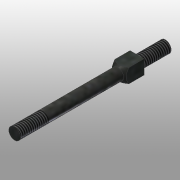
# Autodesk Inventor part: 500-001
Saved by Autodesk Inventor 2016 (Build 200138000, 138)
## iProperties
Created: 2015-04-18
Part Number: 500-001
Material: Steel
Document SubType Name: Modeling
Designer: Station9
Density: 7.85 g/cm^3
Appearance: Plate
Mass: 1.35592 g
Surface Area: 2.8236 cm^2
Volume: 0.172728 cm^3
Author: Station9
Autodesk Inventor part; units mm, degrees
ref_plane "YZ Plane" through (0, 0, 0) normal (1, 0, 0) x (0, 1, 0)
ref_plane "XZ Plane" through (0, 0, 0) normal (0, 1, 0) x (-1, 0, 0)
ref_plane "XY Plane" through (0, 0, 0) normal (0, 0, 1) x (1, 0, 0)
sketch "Sketch1" plane through (0, 0, 0) normal (0, 1, 0) x (-1, 0, 0)
  line L0 (-1.5, 1.5) -> (1.5, 1.5)
  line L1 (1.5, 1.5) -> (1.5, -1.5)
  line L2 (1.5, -1.5) -> (-1.5, -1.5)
  line L3 (-1.5, -1.5) -> (-1.5, 1.5)
  line L4 (-1.5, 1.5) -> (1.5, -1.5) construction
  line L5 (1.5, 1.5) -> (-1.5, -1.5) construction
  point P0 (0, 0)
  dimension "d0" = 3
  dimension "d1" = 3
  constraints: 12 end point, 2 midpoint, 2 parallel, 1 horizontal, 1 perpendicular
  measures "d0" distance of L1.end L2.end
  measures "d1" distance of L0.end L1.end
extrude "Extrusion1" add sketch "Sketch1" along normal blind 4.1
sketch "Sketch2" plane through (0, 4.1, 0) normal (0, 1, 0) x (1, 0, 0)
  circle A0 centre (0, 0) radius 1.25
  dimension "d4" = 2.5
  constraints: 1 centre point, 1 coincident
  measures "d4" diameter of A0
extrude "Extrusion2" add sketch "Sketch2" along normal blind 6
sketch "Sketch3" plane through (0, 0, 0) normal (0, -1, 0) x (1, 0, 0)
  circle A0 centre (0, 0) radius 1.25
  dimension "d7" = 2.5
  constraints: 1 centre point, 1 coincident
  measures "d7" diameter of A0
extrude "Extrusion3" add sketch "Sketch3" along normal blind 21.9
thread "Thread1" size "M2.5x0.45" class "6g" standard "ISO Metric profile" length 6
thread "Thread2" size "M2.5x0.45" class "6g" standard "ISO Metric profile" length 10
sketch "Sketch4" plane through (0, 0, 0) normal (1, 0, 0) x (0, 1, 0)
  line L0 (0, 1.5) -> (4.1, 1.5) construction
  line L1 (4.1, 1.5) -> (4.1, 1.25) construction
  line L2 (4.1, 1.25) -> (10.1, 1.25) construction
  line L3 (10.1, 1.25) -> (10.1, -1.25) construction
  line L4 (10.1, -1.25) -> (4.1, -1.25) construction
  line L5 (4.1, -1.25) -> (4.1, -1.5) construction
  line L6 (4.1, -1.5) -> (0, -1.5) construction
  line L7 (0, -1.5) -> (0, -1.25) construction
  line L8 (0, -1.25) -> (-21.9, -1.25) construction
  line L9 (-21.9, -1.25) -> (-21.9, 1.25) construction
  line L10 (-21.9, 1.25) -> (0, 1.25) construction
  line L11 (0, 1.25) -> (0, 1.5) construction
  line L12 (0, -1.25) -> (0.25, -1.5)
  line L13 (0, -1.25) -> (0.3536, -1.25) construction
  line L14 (0, -1.25) -> (0, -1.5)
  line L15 (0, -1.5) -> (4.1, -1.5) projected
  line L16 (-28.3, 0) -> (16.5, 0) projected
  line L17 (0, -1.5) -> (0, -2.5685)
  line L18 (0, -2.5685) -> (0.9588, -2.2088)
  line L19 (0.9588, -2.2088) -> (0.25, -1.5)
  point P0 (0, 0)
  dimension "d15" = 45
  constraints: 12 end point, 1 collinear, 1 equal length, 1 horizontal, 1 point on line, 1 vertical
  measures "d15" angle of L12 L13
revolve "Revolution1" cut sketch "Sketch4" angle 360 about axis through (0, -10, 0) along (0, 1, 0)
body "Solid1"
